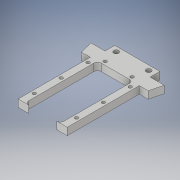
# Autodesk Inventor part: 000.402 - Прижим сервомотора
Saved by Autodesk Inventor 2019 (Build 230136000, 136)
## iProperties
Created: 2020-03-19
Part Number: 000.402 - Прижим сервомотора
Material: Типовые
Document SubType Name: Modeling
Designer: Петров Иван
Density: 1 g/cm^3
Appearance: По умолчанию
Author: Петров Иван
Autodesk Inventor part; units mm, degrees
ref_plane "YZ Plane" through (0, 0, 0) normal (1, 0, 0) x (0, 1, 0)
ref_plane "XZ Plane" through (0, 0, 0) normal (0, 1, 0) x (-1, 0, 0)
ref_plane "XY Plane" through (0, 0, 0) normal (0, 0, 1) x (1, 0, 0)
sketch "Эскиз1" plane through (0, 0, 0) normal (0, 1, 0) x (-1, 0, 0)
  arc A0 (3.5, 65.1) -> (0.5, 62.1) centre (3.5, 62.1) ccw
  line L0 (0, 65.1) -> (3.5, 65.1)
  line L1 (0, 65.1) -> (-5.1, 59.1)
  line L2 (-5.1, 59.1) -> (-5.1, 6)
  line L3 (-5.1, 6) -> (0, 0)
  line L4 (0, 0) -> (30, 0)
  line L5 (30, 0) -> (35.1, 6)
  line L6 (35.1, 6) -> (35.1, 59.1)
  line L7 (35.1, 59.1) -> (30, 65.1)
  line L8 (26.5, 65.1) -> (30, 65.1)
  arc A1 (29.5, 62.1) -> (26.5, 65.1) centre (26.5, 62.1) ccw
  line L9 (29.5, 8.6) -> (29.5, 62.1)
  arc A2 (26.5, 5.6) -> (29.5, 8.6) centre (26.5, 8.6) ccw
  line L10 (3.5, 5.6) -> (26.5, 5.6)
  arc A3 (0.5, 8.6) -> (3.5, 5.6) centre (3.5, 8.6) ccw
  line L11 (0.5, 62.1) -> (0.5, 8.6)
  circle A4 centre (4, 2.8) radius 1.35
  circle A5 centre (-2.3, 10.6) radius 1.35
  circle A6 centre (-2.3, 32.6) radius 1.35
  circle A7 centre (-2.3, 54.6) radius 1.35
  circle A8 centre (26, 2.8) radius 1.35
  circle A9 centre (32.3, 10.6) radius 1.35
  circle A10 centre (32.3, 32.6) radius 1.35
  circle A11 centre (32.3, 54.6) radius 1.35
  line L12 (26.5, 65.1) -> (3.5, 65.1)
  line L13 (35.1, 6) -> (35.1, 0)
  line L14 (35.1, 0) -> (30, 0)
  line L15 (-5.1, 6) -> (-5.1, 0)
  line L16 (-5.1, 0) -> (0, 0)
  line L17 (35.1, 0) -> (-5.1, 0)
  line L18 (-5.1, 0) -> (-5.1, 65.1)
  line L19 (-5.1, 65.1) -> (35.1, 65.1)
  line L20 (35.1, 65.1) -> (35.1, 0)
  point P0 (15, 50.6)
  constraints: 42 end point, 12 centre point, 8 point on circle, 2 parallel, 2 perpendicular, 2 vertical, 1 collinear, 1 horizontal
extrude "Выдавливание1" add sketch "Эскиз1" along normal blind 6 contours A0 L11 A3 L10 A2 L9 A1 L8 L7 L6 L5 L4 L3 L2 L1 L0 | L1 L18 L19 | L19 L20 L7
sketch "Эскиз2" plane through (0, 6, 0) normal (0, 1, 0) x (1, 0, 0)
  circle A0 centre (-1.7123, 8.5046) radius 2
  circle A1 centre (-28.2877, 8.5046) radius 2
  line L0 (3.5, 12.5046) -> (-33.5, 12.5046)
  line L1 (-33.5, 12.5046) -> (-33.5, 4.5046)
  line L2 (-33.5, 4.5046) -> (-45.0593, 4.5046)
  arc A2 (-42.448, -6) -> (-45.0593, 4.5046) centre (-184.8586, -35.8244) ccw
  line L3 (-42.448, -6) -> (-35.1, -6)
  line L4 (-35.1, -6) -> (-30, 0)
  line L5 (-30, 0) -> (0, 0)
  line L6 (0, 0) -> (5.1, -6)
  line L7 (5.1, -6) -> (12.448, -6)
  arc A3 (15.0593, 4.5046) -> (12.448, -6) centre (154.8586, -35.8244) ccw
  line L8 (15.0593, 4.5046) -> (3.5, 4.5046)
  line L9 (3.5, 4.5046) -> (3.5, 12.5046)
  point P0 (0, 0)
  point P1 (0, 0)
  constraints: 20 end point, 4 centre point, 4 point on circle
extrude "Выдавливание2" add sketch "Эскиз2" against normal blind 6
